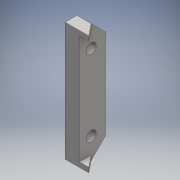
# Autodesk Inventor part: holes
Saved by Autodesk Inventor 2016 (Build 200138000, 138)
## iProperties
Created: 2016-02-09
Part Number: holes
Material: Generic
Document SubType Name: Modeling
Designer: element
Density: 1 g/cm^3
Appearance: Default
Mass: 0.348071 g
Surface Area: 4.77638 cm^2
Volume: 0.348071 cm^3
Author: element
Autodesk Inventor part; units mm, degrees
ref_plane "YZ Plane" through (0, 0, 0) normal (1, 0, 0) x (0, 1, 0)
ref_plane "XZ Plane" through (0, 0, 0) normal (0, 1, 0) x (-1, 0, 0)
ref_plane "XY Plane" through (0, 0, 0) normal (0, 0, 1) x (1, 0, 0)
sketch "Sketch1" plane through (0, 0, 0) normal (1, 0, 0) x (0, 1, 0)
  line L0 (0, 0) -> (0, 8)
  line L1 (0, 8) -> (2.5, 8)
  circle A0 centre (2.5, 8) radius 1.05
  circle A1 centre (2.5, 8) radius 1.9
  dimension "d1" = 8
  dimension "d2" = 2.5
  dimension "d3" = 2.1
  dimension "d7" = 3.8
  constraints: 4 end point, 2 centre point, 2 coincident, 1 horizontal, 1 vertical
  measures "d1" distance of L0.start L0.end
  measures "d2" distance of L0.end L1.end
  measures "d3" diameter of A0
  measures "d7" diameter of A1
sketch "Sketch4" plane through (0, 0, 0) normal (1, 0, 0) x (0, 1, 0)
  line L0 (0, 0) -> (0, 3.5)
  line L1 (0, 3.5) -> (0, 12.5)
  line L2 (0, 12.5) -> (2.5, 12.5)
  line L3 (2.5, 12.5) -> (5.5, 12.5)
  line L4 (5.5, 12.5) -> (5.5, 9.5)
  line L5 (2.5, 12.5) -> (5.5, 9.5)
  line L6 (0, 0) -> (5.5, 0)
  line L7 (5.5, 0) -> (5.5, 9.5)
  dimension "d32" = 3.5
  dimension "d33" = 9
  dimension "d35" = 2.5
  dimension "d37" = 3
  dimension "d38" = 3
  constraints: 16 end point, 3 perpendicular, 2 horizontal, 1 point on line, 1 vertical
  measures "d32" distance of L0.start L0.end
  measures "d33" distance of L0.end L1.end
  measures "d35" distance of L1.end L2.end
  measures "d37" distance of L2.end L3.end
  measures "d38" distance of L3.end L4.end
extrude "Extrusion3" add sketch "Sketch4" along normal blind 3 contours L0 L1 L2 L5 L7 L6
sketch "Sketch9" plane through (3, 0, 0) normal (1, 0, 0) x (0, 0, -1)
  line L0 (0, 0) -> (-3.5, 0)
  line L1 (-12.5, 0) -> (0, 0) projected
  line L2 (-3.5, 0) -> (-4.5, 0)
  line L3 (-3.5, 0) -> (-3.5, 2.5)
  line L4 (-3.5, 2.5) -> (-4.5, 2.5)
  line L5 (-4.5, 2.5) -> (-4.5, 0)
  line L6 (-4.5, 0) -> (-11.5, 0)
  line L7 (-11.5, 2.5) -> (-12.5, 2.5)
  line L8 (-11.5, 2.5) -> (-11.5, 0)
  line L9 (-12.5, 2.5) -> (-12.5, 0)
  line L10 (-12.5, 0) -> (-11.5, 0)
  dimension "d70" = 3.5
  dimension "d71" = 1
  dimension "d72" = 1
  dimension "d73" = 7
  dimension "d74" = 2.5
  constraints: 20 end point, 4 point on line, 3 vertical, 2 perpendicular, 1 collinear, 1 horizontal
  measures "d70" distance of L0.start L0.end
  measures "d71" distance of L3.end L4.end
  measures "d72" distance of L7.start L7.end
  measures "d73" distance between parallel lines of L5 L8
  measures "d74" distance of L0.end L3.end
extrude "Extrusion4" add sketch "Sketch9" along normal blind 2 contours L9 L7 L8 L1
sketch "Sketch10" plane through (0, 0, 12.5) normal (0, 0, 1) x (1, 0, 0)
  line L0 (3, 0) -> (3, 5.5) projected
  line L1 (3, 0) -> (5, 0)
  line L2 (3, 0) -> (3, 2.5)
  line L3 (3, 2.5) -> (5, 2.5)
  line L4 (5, 2.5) -> (5, 0)
  line L5 (3, 2.5) -> (5, 0)
  point P0 (0, 0)
  dimension "d110" = 2
  dimension "d111" = 2.5
  constraints: 10 end point, 2 horizontal, 1 perpendicular, 1 point on line
  measures "d110" distance of L0.start L1.end
  measures "d111" distance of L0.start L2.end
extrude "Extrusion9" cut sketch "Sketch10" against normal blind 1 contours L3 L4 L5
hole "Hole5" at (0, 2.5, 8) direction (1, 0, 0) diameter 3.8 depth 1.2
hole "Hole6" at (0, 2.5, 8) direction (1, 0, 0) diameter 2.1 end through all
mirror "Mirror3" about plane through (0, 0, 0) normal (0, 0, 1) of "Extrusion3", "Extrusion4", "Extrusion9", "Hole5", "Hole6"
equation "\"d38\" = d37"
equation "\"d90\" = d7"
equation "\"d97\" = d3"
body "Solid3"
